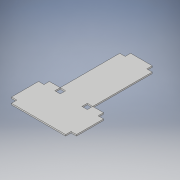
# Autodesk Inventor part: BT003_trajan20_21
Saved by Autodesk Inventor 2022.2 (Build 262287000, 287)
## iProperties
Company: HTBLA Kaindorf
RuleStatus: InUse
Created: 2022-08-03
Part Number: BT003_trajan20_21
Project: Zeichenmaschine_v2
Material: Generisch
Description: Platte unten
Document SubType Name: Modeling
Designer: trajan20
Density: 1 g/cm^3
Appearance: Vorgabe
Mass: 296 g
Surface Area: 1254 cm^2
Volume: 296 cm^3
AfterDocNew0: iProperties-Editor_aufrufen
Author: jan
Keywords: 2021
Autodesk Inventor part; units mm, degrees
ref_plane "YZ Plane" through (0, 0, 0) normal (1, 0, 0) x (0, 1, 0)
ref_plane "XZ Plane" through (0, 0, 0) normal (0, 1, 0) x (-1, 0, 0)
ref_plane "XY Plane" through (0, 0, 0) normal (0, 0, 1) x (1, 0, 0)
sketch "Skizze3" plane through (0, 0, 0) normal (0, 0, 1) x (1, 0, 0)
  line L0 (0, 0) -> (0, 200)
  line L1 (0, 200) -> (-20, 200)
  line L2 (-20, 200) -> (-20, 220)
  line L3 (-20, 220) -> (-120, 220)
  line L4 (-120, 220) -> (-120, 200)
  line L5 (-120, 200) -> (-140, 200)
  line L6 (-140, 200) -> (-140, 160)
  line L7 (-140, 160) -> (-120, 160)
  line L8 (-120, 160) -> (-120, 140)
  line L9 (-120, 140) -> (-140, 140)
  line L10 (-140, 140) -> (-140, 160)
  line L11 (-140, 160) -> (-360, 160)
  line L12 (-360, 160) -> (-360, 140)
  line L13 (-360, 140) -> (-380, 140)
  line L14 (-380, 140) -> (-380, 60)
  line L15 (-380, 60) -> (-360, 60)
  line L16 (-360, 60) -> (-360, 40)
  line L17 (-360, 40) -> (-140, 40)
  line L18 (-140, 40) -> (-140, 60)
  line L19 (-140, 60) -> (-120, 60)
  line L20 (-120, 60) -> (-120, 40)
  line L21 (-120, 40) -> (-140, 40)
  line L22 (-140, 40) -> (-140, 0)
  line L23 (-140, 0) -> (-120, 0)
  line L24 (-120, 0) -> (-120, -20)
  line L25 (-120, -20) -> (-20, -20)
  line L26 (-20, -20) -> (-20, 0)
  line L27 (-20, 0) -> (0, 0)
  dimension "d4" = 200
  dimension "d5" = 20
  dimension "d6" = 20
  dimension "d7" = 100
  dimension "d8" = 20
  dimension "d9" = 20
  dimension "d10" = 20
  dimension "d11" = 40
  dimension "d12" = 220
  dimension "d13" = 20
  dimension "d14" = 20
  dimension "d15" = 220
  dimension "d16" = 80
  dimension "d17" = 20
  dimension "d18" = 20
  dimension "d19" = 20
  dimension "d20" = 100
  dimension "d21" = 20
  dimension "d22" = 20
  dimension "d23" = 40
  constraints: 56 end point, 18 perpendicular, 6 point on line, 5 vertical, 2 horizontal
  measures "d4" distance of L0.start L0.end
  measures "d5" distance of L0.end L1.end
  measures "d6" distance of L1.end L2.end
  measures "d7" distance of L2.end L3.end
  measures "d8" distance of L4.end L5.end
  measures "d9" distance between parallel lines of L9 L7
  measures "d10" distance between parallel lines of L10 L8
  measures "d11" distance of L5.end L6.end
  measures "d12" distance of L6.end L11.end
  measures "d13" distance between parallel lines of L14 L12
  measures "d14" distance of L15.end L16.end
  measures "d15" distance of L16.end L17.end
  measures "d16" distance between parallel lines of L15 L13
  measures "d17" distance between parallel lines of L14 L16
  measures "d18" distance of L25.end L26.end
  measures "d19" distance of L22.end L23.end
  measures "d20" distance of L24.end L25.end
  measures "d21" distance between parallel lines of L18 L20
  measures "d22" distance of L19.end L20.end
  measures "d23" distance of L17.end L22.end
extrude "Extrusion3" add sketch "Skizze3" along normal blind 5
